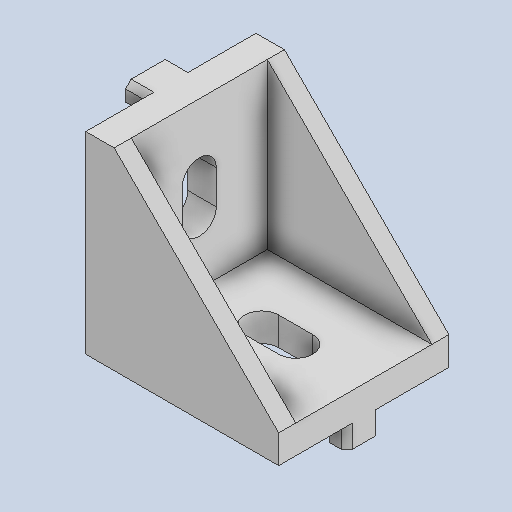
# Autodesk Inventor part: L
Saved by Autodesk Inventor 2025 (Build 290162000, 162)
## iProperties
Created: 2025-09-03
Part Number: L
Material: Generic
Document SubType Name: Modeling
Designer: Pravoslav
Density: 1 g/cm^3
Appearance: Default
Author: Pravoslav
Autodesk Inventor part; units mm, degrees
ref_plane "YZ Plane" through (0, 0, 0) normal (1, 0, 0) x (0, 1, 0)
ref_plane "XZ Plane" through (0, 0, 0) normal (0, 1, 0) x (-1, 0, 0)
ref_plane "XY Plane" through (0, 0, 0) normal (0, 0, 1) x (1, 0, 0)
sketch "Sketch1" plane through (0, 0, 0) normal (0, 1, 0) x (-1, 0, 0)
  line L0 (17, 15) -> (-17, 15)
  line L1 (-17, 15) -> (-17, -15)
  line L2 (-17, -15) -> (17, -15)
  line L3 (17, -15) -> (17, 15)
  line L4 (17, 15) -> (-17, -15) construction
  line L5 (-17, 15) -> (17, -15) construction
  circle A0 centre (-5, 0) radius 3
  circle A1 centre (1, 0) radius 3
  line L6 (1, 3) -> (-5, 3)
  line L7 (1, -3) -> (-5, -3)
  point P0 (0, 0)
  dimension "d0" = 34
  dimension "d1" = 30
  dimension "d2" = 6
  dimension "d3" = 12
  dimension "d4" = 6
  dimension "d5" = 18
  constraints: 16 end point, 4 point on circle, 3 parallel, 2 centre point, 2 horizontal, 2 midpoint, 1 perpendicular, 1 tangent
  measures "d0" distance of L2.end L1.end
  measures "d1" distance of L1.end L0.end
  measures "d2" diameter of A0
  measures "d3" distance from line of L1 A0.centre
  measures "d4" diameter of A1
  measures "d5" distance from line of L1 A1.centre
extrude "Extrusion1" add sketch "Sketch1" along normal blind 5
sketch "Sketch2" plane through (-17, 0, -15) normal (-1, 0, 0) x (0, 0, 1)
  line L0 (30, 0) -> (0, 0) projected
  line L1 (0, 0) -> (30, 0)
  line L2 (30, 0) -> (30, 34)
  line L3 (30, 34) -> (0, 34)
  line L4 (0, 34) -> (0, 0)
  circle A0 centre (15, 16) radius 3
  circle A1 centre (15, 22) radius 3
  line L5 (12, 22) -> (12, 16)
  line L6 (18, 22) -> (18, 16)
  point P0 (15, 0)
  point P1 (15, 0)
  dimension "d8" = 34
  dimension "d9" = 6
  dimension "d10" = 6
  dimension "d11" = 0
  dimension "d12" = 0
  dimension "d13" = 6
  dimension "d15" = 12
  constraints: 12 end point, 4 point on circle, 3 parallel, 2 centre point, 1 horizontal, 1 midpoint, 1 perpendicular, 1 tangent, 1 vertical
  measures "d8" distance of L2.end L1.end
  measures "d9" diameter of A0
  measures "d10" diameter of A1
  measures "d11" horizontal distance of A0.centre A1.centre
  measures "d12" horizontal distance of point (15, 0) A0.centre
  measures "d13" distance of A1.centre A0.centre
  measures "d15" distance from line of L3 A1.centre
extrude "Extrusion2" add sketch "Sketch2" against normal blind 5
sketch "Sketch3" plane through (17, 0, -15) normal (0, 0, -1) x (-1, 0, 0)
  line L0 (34, 34) -> (29, 34) projected
  line L1 (0, 5) -> (29, 34)
  line L2 (29, 34) -> (29, 5)
  line L3 (29, 5) -> (0, 5)
  point P0 (17, 0)
  constraints: 6 end point, 2 perpendicular
extrude "Extrusion3" add sketch "Sketch3" against normal blind 3
mirror "Mirror1" about plane through (0, 0, 0) normal (0, 0, 1) of "Extrusion3"
sketch "Sketch4" plane through (0, 0, 0) normal (0, -1, 0) x (1, 0, 0)
  line L0 (20, 3) -> (14, 3)
  line L1 (14, 3) -> (14, -3)
  line L2 (14, -3) -> (20, -3)
  line L3 (20, -3) -> (20, 3)
  line L4 (17, 15) -> (17, -15) projected
  line L5 (20, 3) -> (14, -3) construction
  line L6 (14, 3) -> (20, -3) construction
  line L7 (17, 3) -> (17, -3)
  line L8 (-20, 3) -> (-14, 3)
  line L9 (-14, 3) -> (-14, -3)
  line L10 (-14, -3) -> (-20, -3)
  line L11 (-20, -3) -> (-20, 3)
  line L12 (-17, -3) -> (-17, 3) projected
  line L13 (-20, 3) -> (-14, -3) construction
  line L14 (-14, 3) -> (-20, -3) construction
  line L15 (-17, 3) -> (-17, -3)
  line L16 (-17, -15) -> (-17, 15) projected
  point P0 (0, 0)
  point P1 (17, 0)
  point P2 (-17, 0)
  dimension "d20" = 6
  dimension "d21" = 6
  dimension "d22" = 6
  dimension "d23" = 6
  constraints: 28 end point, 8 midpoint, 4 parallel, 2 horizontal, 2 perpendicular, 2 point on line, 1 collinear
  measures "d20" distance of L2.end L1.end
  measures "d21" distance of L1.end L0.end
  measures "d22" distance of L9.end L10.end
  measures "d23" distance of L8.end L9.end
extrude "Extrusion4" add sketch "Sketch4" along normal blind 4 contours L4 L2 L1 L0 | L8 L9 L10 L12
chamfer "Chamfer1" distance 1 angle 45 4 edges at (17, -2, 3) (17, -2, -3) (-17, -2, -3) (-17, -2, 3)
sketch "Sketch5" plane through (-17, 34, -15) normal (-1, 0, 0) x (0, 0, 1)
  line L0 (11, 3) -> (19, 3)
  line L1 (19, 3) -> (19, -3)
  line L2 (19, -3) -> (11, -3)
  line L3 (11, -3) -> (11, 3)
  line L4 (30, 0) -> (0, 0) projected
  line L5 (11, 3) -> (19, -3) construction
  line L6 (19, 3) -> (11, -3) construction
  line L7 (11, -31) -> (19, -31)
  line L8 (19, -31) -> (19, -37)
  line L9 (19, -37) -> (11, -37)
  line L10 (11, -37) -> (11, -31)
  line L11 (11, -31) -> (19, -37) construction
  line L12 (19, -31) -> (11, -37) construction
  line L13 (11, 0) -> (19, 0)
  line L14 (0, -34) -> (13, -34) projected
  line L15 (11, -34) -> (19, -34)
  point P0 (15, -34)
  point P1 (15, 0)
  dimension "d29" = 8
  dimension "d30" = 6
  dimension "d31" = 8
  dimension "d32" = 6
  constraints: 28 end point, 9 midpoint, 4 parallel, 3 point on line, 2 horizontal, 2 perpendicular
  measures "d29" distance of L1.end L2.end
  measures "d30" distance of L0.end L1.end
  measures "d31" distance of L8.end L9.end
  measures "d32" distance of L7.end L8.end
extrude "Extrusion5" add sketch "Sketch5" along normal blind 4 contours L4 L1 L2 L3 | L7 L8 L15 L14 L10
chamfer "Chamfer2" distance 1 angle 45 4 edges at (-19, 0, -4) (-19, 0, 4) (-19, 34, 4) (-19, 34, -4)
body "Solid1"
